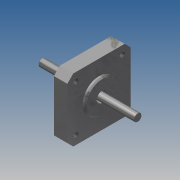
# Autodesk Inventor part: Frontplatte
Saved by Autodesk Inventor 2015 (Build 190159000, 159)
## iProperties
Created: 2015-01-06
Part Number: Frontplatte
Material: Stahl, Kohlenstoff
Document SubType Name: Modeling
Designer: Marc
Density: 7.85 g/cm^3
Appearance: Halbpoliert
Mass: 71.3616 g
Surface Area: 46.3336 cm^2
Volume: 9.09064 cm^3
Author: Marc
Autodesk Inventor part; units mm, degrees
ref_plane "YZ Plane" through (0, 0, 0) normal (1, 0, 0) x (0, 1, 0)
ref_plane "XZ Plane" through (0, 0, 0) normal (0, 1, 0) x (-1, 0, 0)
ref_plane "XY Plane" through (0, 0, 0) normal (0, 0, 1) x (1, 0, 0)
sketch "Skizze1" plane through (0, 0, 0) normal (1, 0, 0) x (0, 1, 0)
  line L0 (-29.61, 0) -> (29.61, 0) projected
  line L1 (0, -29.61) -> (0, 29.61) projected
  line L2 (-17.15, 21.15) -> (17.15, 21.15)
  line L3 (21.15, 17.15) -> (21.15, -17.15)
  line L4 (17.15, -21.15) -> (-17.15, -21.15)
  line L5 (-21.15, -17.15) -> (-21.15, 17.15)
  line L6 (21.15, 17.15) -> (17.15, 21.15)
  line L7 (21.15, -17.15) -> (17.15, -21.15)
  line L8 (-17.15, -21.15) -> (-21.15, -17.15)
  line L9 (-17.15, 21.15) -> (-21.15, 17.15)
  circle A0 centre (0, 0) radius 3.5
  point P0 (-21.15, 21.15)
  point P1 (21.15, -21.15)
  point P2 (21.15, 21.15)
  point P3 (-21.15, -21.15)
  dimension "d0" = 42.3
  dimension "d1" = 42.3
  dimension "d5" = 4
  dimension "d6" = 4
  dimension "d7" = 4
  dimension "d8" = 4
  dimension "d9" = 4
  dimension "d10" = 4
  dimension "d11" = 4
  dimension "d12" = 4
  dimension "d13" = 7
  constraints: 16 end point, 8 point on line, 2 parallel, 1 centre point, 1 coincident, 1 horizontal, 1 perpendicular, 2 other
  measures "d0" distance of point (21.15, -21.15) point (-21.15, -21.15)
  measures "d1" distance of point (21.15, 21.15) point (21.15, -21.15)
  measures "d5" distance of L3.start point (21.15, 21.15)
  measures "d6" distance of L2.end point (21.15, 21.15)
  measures "d7" distance of L3.end point (21.15, -21.15)
  measures "d8" distance of L4.start point (21.15, -21.15)
  measures "d9" distance of L4.end point (-21.15, -21.15)
  measures "d10" distance of L5.start point (-21.15, -21.15)
  measures "d11" distance of L2.start point (-21.15, 21.15)
  measures "d12" distance of L5.end point (-21.15, 21.15)
  measures "d13" diameter of A0
extrude "Extrusion2" add sketch "Skizze1" along normal mid plane 9 contours L5 L9 L2 L1 A0 L0 | L0 A0 L1 L4 L8 L5 | L1 L2 L6 L3 L0 A0 | A0 L0 L3 L7 L4 L1
sketch "Skizze2" plane through (4.5, 0, 0) normal (1, 0, 0) x (0, 0, -1)
  circle A0 centre (0, 0) radius 3.5 projected
  line L0 (-17.15, 21.15) -> (-21.15, 17.15) projected
  line L1 (-21.15, 17.15) -> (-21.15, -17.15) projected
  line L2 (-21.15, -17.15) -> (-17.15, -21.15) projected
  line L3 (-17.15, -21.15) -> (17.15, -21.15) projected
  line L4 (17.15, -21.15) -> (21.15, -17.15) projected
  line L5 (21.15, -17.15) -> (21.15, 17.15) projected
  line L6 (21.15, 17.15) -> (17.15, 21.15) projected
  line L7 (17.15, 21.15) -> (-17.15, 21.15) projected
  line L8 (0, -29.61) -> (0, 29.61) projected
  line L9 (29.61, 0) -> (-29.61, 0) projected
  point P0 (-15.5, 15.5)
  point P1 (15.5, 15.5)
  point P2 (-15.5, -15.5)
  point P3 (15.5, -15.5)
  dimension "d18" = 15.5
  dimension "d19" = 15.5
  constraints: 3 symmetric about line
  measures "d18" distance from line of L9 point (-15.5, 15.5)
  measures "d19" distance from line of L8 point (-15.5, 15.5)
hole "Bohrung1" at (4.5, 15.5, 15.5) at (4.5, 15.5, -15.5) at (4.5, -15.5, 15.5) at (4.5, -15.5, -15.5) direction (-1, 0, 0) diameter 3.242 end through all thread size "M4x0.7" class "6H" standard "ISO Metric profile"
sketch "Skizze3" plane through (4.5, 0, 0) normal (1, 0, 0) x (0, 0, -1)
  line L0 (0, -29.61) -> (0, 29.61) projected
  line L1 (29.61, 0) -> (-29.61, 0) projected
  circle A0 centre (0, 0) radius 11
  circle A1 centre (0, 0) radius 3.5
  dimension "d27" = 22
  dimension "d28" = 7
  constraints: 2 centre point, 2 coincident
  measures "d27" diameter of A0
  measures "d28" diameter of A1
extrude "Extrusion3" add sketch "Skizze3" along normal blind 2 contours A0 L1 A1 L0 | L0 A1 L1 A0 | A0 L0 A1 L1 | L1 A1 L0 A0
chamfer "Fase1" distance 0.8 angle 45 1 edges at (6.5, 0, 11)
sketch "Skizze4" plane through (6.5, 0, 0) normal (1, 0, 0) x (0, 0, -1)
  line L0 (29.61, 0) -> (-29.61, 0) projected
  line L1 (0, -29.61) -> (0, 29.61) projected
  circle A0 centre (0, 0) radius 2.5
  dimension "d34" = 5
  constraints: 1 centre point, 1 coincident
  measures "d34" diameter of A0
extrude "Extrusion4" add sketch "Skizze4" along normal blind 24 and the other way blind 40
chamfer "Fase2" distance 0.2 angle 45 1 edges at (30.5, 0, 2.5)
chamfer "Fase3" distance 0.2 angle 45 1 edges at (-33.5, 0, 2.5)
equation "\"d6\" = d5"
equation "\"d8\" = d7"
equation "\"d9\" = d7"
equation "\"d10\" = d9"
equation "\"d11\" = d7"
equation "\"d12\" = d11"
